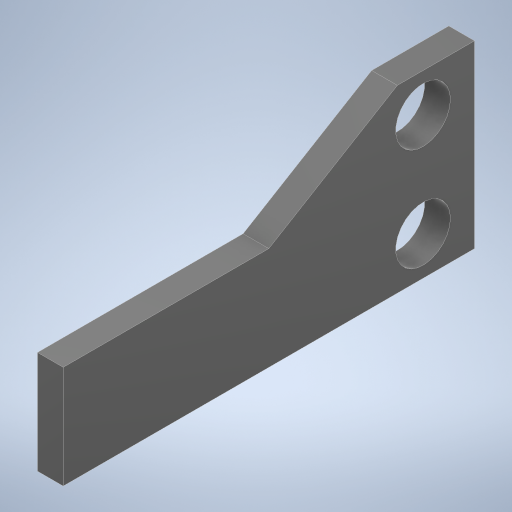
# Autodesk Inventor part: Carriage
Saved by Autodesk Inventor 2024 (Build 280153000, 153)
## iProperties
Created: 2023-12-18
Part Number: Carriage
Material: Generic
Document SubType Name: Modeling
Designer: greg
Density: 1 g/cm^3
Appearance: Smooth - Black
Author: greg
Autodesk Inventor part; units mm, degrees
ref_plane "YZ Plane" through (0, 0, 0) normal (1, 0, 0) x (0, 1, 0)
ref_plane "XZ Plane" through (0, 0, 0) normal (0, 1, 0) x (-1, 0, 0)
ref_plane "XY Plane" through (0, 0, 0) normal (0, 0, 1) x (1, 0, 0)
sketch "Sketch1" plane through (0, 0, 0) normal (1, 0, 0) x (0, 1, 0)
  line L0 (12.7, 50.8) -> (0, 50.8)
  line L1 (0, 50.8) -> (0, 0)
  circle A0 centre (4.7625, 6.35) radius 1.27
  circle A1 centre (17.4625, 6.35) radius 1.27
  line L2 (12.7, 50.8) -> (12.7, 25.4)
  line L3 (12.7, 25.4) -> (22.225, 9.525)
  line L4 (22.225, 9.525) -> (22.225, 0)
  line L5 (17.4625, 6.35) -> (4.7625, 6.35) construction
  line L6 (22.225, 0) -> (0, 0)
  circle A2 centre (17.4625, 6.35) radius 3.81 construction
  circle A3 centre (4.7625, 6.35) radius 3.81 construction
  point P0 (11.1125, 6.35)
  point P1 (11.1125, 0)
  dimension "d0" = 12.7
  dimension "d2" = 2.54
  dimension "d4" = 12.7
  dimension "d5" = 9.525
  dimension "d6" = 15.875
  dimension "d7" = 50.8
  dimension "d8" = 22.225
  dimension "d9" = 6.35
  dimension "d10" = 7.62
  constraints: 14 end point, 4 centre point, 2 coincident, 2 equal radius, 2 horizontal, 2 midpoint, 2 vertical, 1 parallel, 1 perpendicular, 1 vertical alignment
  measures "d0" distance of L0.end L0.start
  measures "d2" diameter of A0
  measures "d4" distance of L5.end L5.start
  measures "d5" distance of L3.end L4.end
  measures "d6" vertical distance of L2.end L3.end
  measures "d7" distance of L0.end L1.end
  measures "d8" distance of L4.end L1.end
  measures "d9" distance from line of point (11.113, 0) L5
  measures "d10" diameter of A2
extrude "Extrusion1" add sketch "Sketch1" along normal blind 3.175
sketch "Sketch2" plane through (3.175, 0, 0) normal (1, 0, 0) x (0, 0, -1)
  circle A0 centre (-6.35, 17.4625) radius 1.27 projected
  circle A1 centre (-6.35, 4.7625) radius 1.27 projected
  point P0 (0, 0)
  constraints: 2 coincident
hole "Hole1" at (3.175, 17.4625, 6.35) at (3.175, 4.7625, 6.35) direction (-1, 0, 0) diameter 6.7564 end through all clearance for "Flat Head Machine Screw (82)" size "1/4" standard "Ansi Unified Screw Threads"
body "Solid1"
